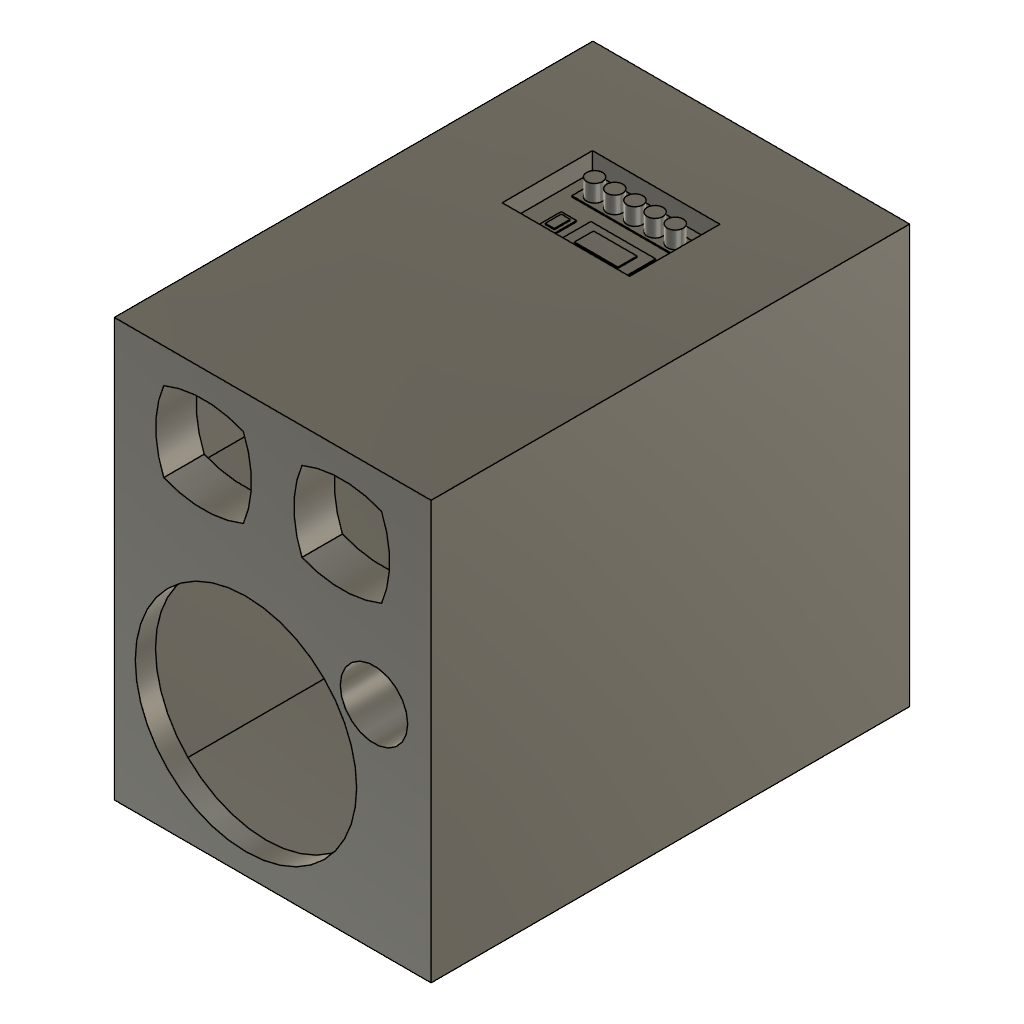
Speaker (Autodesk Fusion 360 design; units mm, degrees)
Autodesk Fusion 360 part; units mm, degrees
sketch "Sketch1" plane through (0, 0, 0) normal (0, 0, 1) x (1, 0, 0)
  line L0 (0, 0) -> (298.45, 0)
  line L1 (298.45, 0) -> (298.45, 450.85)
  line L2 (298.45, 450.85) -> (0, 450.85)
  line L3 (0, 450.85) -> (0, 0)
  dimension "d1" = 298.45
  dimension "d2" = 450.85
  constraint horizontal L0
  constraint vertical L1
  constraint horizontal L2
  constraint vertical L3
  constraint coincident L0.start L3.end
  measures "d1" distance of L0.start L0.end
  measures "d2" distance of L0.start L2.end
extrude "Extrude1" add sketch "Sketch1" along normal blind 254 makes body 1
sketch "Sketch2" plane through (0, 0, 0) normal (0, -1, 0) x (1, 0, 0)
  line L0 (0, 0) -> (298.45, 0)
  line L1 (298.45, 0) -> (298.45, 254)
  line L2 (298.45, 254) -> (0, 254)
  line L3 (0, 254) -> (0, 0)
  line L4 (19.05, 19.05) -> (279.4, 19.05)
  line L5 (279.4, 19.05) -> (279.4, 234.95)
  line L6 (279.4, 234.95) -> (19.05, 234.95)
  line L7 (19.05, 234.95) -> (19.05, 19.05)
  circle A0 centre (124.05, 124.05) radius 104.25
  circle A1 centre (244.65, 200.2) radius 31.75
  circle A2 centre (244.65, 200.2) radius 34.75
  dimension "d5" = -19.05
  dimension "d6" = 208.5
  dimension "d7" = 105
  dimension "d8" = 105
  dimension "d9" = 63.5
  dimension "d10" = 34.75
  dimension "d11" = 34.75
  dimension "d12" = 3
  measures "d6" diameter of A0
  measures "d7" distance of L7 A0.centre
  measures "d8" distance of L4 A0.centre
  measures "d9" diameter of A1
  measures "d10" distance of L5 A1.centre
  measures "d11" distance of L6 A1.centre
extrude "Extrude2" add 1 faces at (99.4833, 150.2833, 254) along direction (0, 0, 1) blind 139.7 on bodies 1 bodies 1
sketch "Sketch3" plane through (0, 0, 0) normal (0, -1, 0) x (1, 0, 0)
  line L0 (0, 0) -> (298.45, 0)
  line L1 (298.45, 0) -> (298.45, 393.7)
  line L2 (298.45, 393.7) -> (0, 393.7)
  line L3 (0, 393.7) -> (0, 0)
  line L4 (298.45, 254) -> (0, 254)
  line L5 (0, 393.7) -> (298.45, 393.7)
  line L6 (298.45, 393.7) -> (298.45, 254)
  line L7 (298.45, 254) -> (0, 254)
  line L8 (0, 254) -> (0, 393.7)
  line L9 (279.4, 273.05) -> (19.05, 273.05)
  line L10 (19.05, 273.05) -> (19.05, 374.65)
  line L11 (19.05, 374.65) -> (279.4, 374.65)
  line L12 (279.4, 374.65) -> (279.4, 273.05)
  line L13 (46.6375, 361.35) -> (121.6375, 361.35)
  line L14 (121.6375, 361.35) -> (121.6375, 286.35)
  line L15 (121.6375, 286.35) -> (46.6375, 286.35)
  line L16 (46.6375, 286.35) -> (46.6375, 361.35)
  line L17 (84.1375, 361.35) -> (84.1375, 340.8281)
  line L18 (19.05, 374.65) -> (149.225, 374.65)
  line L19 (149.225, 374.65) -> (279.4, 374.65)
  line L20 (46.6375, 323.85) -> (54.2725, 323.85)
  line L21 (149.225, 374.65) -> (149.225, 361.3588)
  arc A0 (121.6375, 361.35) -> (46.6375, 361.35) centre (84.1375, 271.8919) ccw
  arc A1 (46.6375, 286.35) -> (121.6375, 286.35) centre (84.1375, 375.8081) ccw
  arc A2 (121.6375, 286.35) -> (121.6375, 361.35) centre (32.1794, 323.85) ccw
  arc A3 (46.6375, 361.35) -> (46.6375, 286.35) centre (136.0956, 323.85) ccw
  arc A4 (251.8125, 361.35) -> (176.8125, 361.35) centre (214.3125, 271.8919) ccw
  arc A5 (176.8125, 361.35) -> (176.8125, 286.35) centre (266.2706, 323.85) ccw
  arc A6 (176.8125, 286.35) -> (251.8125, 286.35) centre (214.3125, 375.8081) ccw
  arc A7 (251.8125, 286.35) -> (251.8125, 361.35) centre (162.3544, 323.85) ccw
  dimension "d15" = 19.05
  dimension "d16" = 75
  dimension "d17" = 75
  dimension "d18" = 65.0875
  dimension "d19" = 50.8
  dimension "d20" = 97
  dimension "d21" = 97
  dimension "d22" = 97
  dimension "d23" = 97
  constraint horizontal L5
  constraint vertical L6
  constraint horizontal L7
  constraint vertical L8
  constraint coincident L4.start L6.end
  constraint coincident L2.end L3.start
  constraint horizontal L13
  constraint vertical L14
  constraint horizontal L15
  constraint vertical L16
  constraint midpoint L13 L17.start
  constraint perpendicular L13 L17
  constraint midpoint L11 L18.end
  constraint midpoint L16 L20.start
  constraint perpendicular L16 L20
  constraint perpendicular L11 L21
  constraint symmetric L13.start L21 A4.start
  constraint symmetric L13.end L21 A4.end
  constraint symmetric L14.end L21 A5.end
  constraint symmetric L15.end L21 A6.end
  constraint symmetric L21 A0 A4
  constraint symmetric L21 A1 A6
  constraint symmetric L21 A2 A5
  constraint symmetric L21 A3 A7
  measures "d16" distance of L13.start L13.end
  measures "d17" distance of L13.start L15.end
  measures "d18" distance of L10 L17
  measures "d19" distance of L18 L20
  measures "d20" radius of A0
  measures "d21" radius of A2
  measures "d22" radius of A1
  measures "d23" radius of A3
extrude "Extrude3" cut sketch "Sketch3" sketch "Sketch2" against normal blind 19.05 contours L13 A0 | L13 L14 L15 L16 | L16 A3 | L14 A2 | L15 A1 | A4 A5 A6 A7 of sketch 2 contours A0 bodies 1
shell "Shell1" thickness 19.05 removed faces 1 at (78.1482, 19.05, 149.2169) on bodies 1
extrude "Extrude4" cut 1 faces at (69.1235, 19.05, 323.85) along direction (0, 1, 0) blind 45 on bodies 1 bodies 1
extrude "Extrude5" cut 1 faces at (214.3125, 19.05, 308.836) along direction (0, 1, 0) blind 95 on bodies 1 bodies 1
extrude "Extrude6" add sketch "Sketch2" against normal blind 314.96 contours A2 | A1 bodies 1
extrude "Extrude7" cut sketch "Sketch2" against normal blind 325 contours A1 bodies 1
sketch "Sketch4" plane through (298.45, 0, 0) normal (1, 0, 0) x (0, 1, 0)
  line L0 (0, 0) -> (450.85, 0)
  line L1 (450.85, 0) -> (450.85, 393.7)
  line L2 (450.85, 393.7) -> (0, 393.7)
  line L3 (0, 393.7) -> (0, 0)
  line L4 (0, 254) -> (263.525, 254)
  line L5 (263.525, 254) -> (450.85, 254)
  line L6 (450.85, 254) -> (450.85, 393.7)
  line L7 (450.85, 393.7) -> (263.525, 393.7)
  line L8 (263.525, 393.7) -> (263.525, 254)
  point P0 (0, 254)
  dimension "d35" = 263.525
  constraint coincident P0 L4.start
  constraint perpendicular L3 L4
  constraint horizontal L5
  constraint vertical L6
  constraint horizontal L7
  constraint vertical L8
  constraint coincident L1.end L2.start
  measures "d35" distance of P0 L4.end
extrude "Extrude8" cut sketch "Sketch4" against normal blind 390 contours L1 L2 L5 L6 L7 L8 bodies 1
sketch "Sketch5" plane through (0, 450.85, 0) normal (0, 1, 0) x (-1, 0, 0)
  line L0 (0, 254) -> (-298.45, 254)
  line L1 (-298.45, 254) -> (-298.45, 0)
  line L2 (-298.45, 0) -> (0, 0)
  line L3 (0, 0) -> (0, 254)
  line L4 (-298.45, 254) -> (0, 254)
  line L5 (0, 254) -> (0, 234.95)
  line L6 (0, 234.95) -> (-298.45, 234.95)
  line L7 (-298.45, 234.95) -> (-298.45, 254)
  dimension "d38" = 19.05
  constraint horizontal L4
  constraint vertical L5
  constraint horizontal L6
  constraint vertical L7
  constraint coincident L0.end L1.start
  measures "d38" distance of L0.end L6.end
extrude "Extrude9" add sketch "Sketch5" against normal blind 450 contours L0 L1 L3 L4 L5 L6 L7 bodies 1
sketch "Sketch6" plane through (0, 0, 393.7) normal (0, 0, 1) x (-1, 0, 0)
  line L0 (-298.45, -263.525) -> (0, -263.525)
  line L1 (0, -263.525) -> (0, 0)
  line L2 (0, 0) -> (-298.45, 0)
  line L3 (-298.45, 0) -> (-298.45, -263.525)
  line L4 (0, -263.525) -> (-298.45, -263.525)
  line L5 (-298.45, -263.525) -> (-298.45, -244.475)
  line L6 (-298.45, -244.475) -> (0, -244.475)
  line L7 (0, -244.475) -> (0, -263.525)
  dimension "d41" = 19.05
  constraint horizontal L4
  constraint vertical L5
  constraint horizontal L6
  constraint vertical L7
  constraint coincident L0.end L1.start
  measures "d41" distance of L0.end L6.end
extrude "Extrude10" add sketch "Sketch6" against normal blind 140 contours L0 L1 L3 L4 L5 L6 L7 bodies 1
sketch "Battery" plane through (0, 0, 254) normal (0, 0, 1) x (-1, 0, 0)
  line L0 (0, -263.525) -> (-298.45, -263.525)
  line L1 (-298.45, -263.525) -> (-298.45, -450.85)
  line L2 (-298.45, -450.85) -> (0, -450.85)
  line L3 (0, -450.85) -> (0, -263.525)
  line L4 (-217.7141, -363.1024) -> (-80.7141, -363.1024)
  line L5 (-80.7141, -363.1024) -> (-80.7141, -429.8524)
  line L6 (-80.7141, -429.8524) -> (-217.7141, -429.8524)
  line L7 (-217.7141, -429.8524) -> (-217.7141, -363.1024)
  line L8 (-198.0587, -450.85) -> (-198.0587, -431.8)
  dimension "d44" = 137
  dimension "d45" = 66.75
  dimension "d100" = 19.05
  constraint horizontal L4
  constraint vertical L5
  constraint horizontal L6
  constraint vertical L7
  constraint coincident L2 L8.start
  constraint perpendicular L2 L8
  measures "d44" distance of L4.start L4.end
  measures "d45" distance of L4.start L6.end
  measures "d100" distance of L8.start L8.end
extrude "Extrude11" add sketch "Battery" along normal blind 82 separate body contours L4 L5 L6 L7 makes body 2
sketch "Sketch8" plane through (0, 0, 254) normal (0, 0, 1) x (-1, 0, 0)
  line L0 (0, -263.525) -> (-298.45, -263.525)
  line L1 (-298.45, -263.525) -> (-298.45, -450.85)
  line L2 (-298.45, -450.85) -> (0, -450.85)
  line L3 (0, -450.85) -> (0, -263.525)
  line L4 (-298.45, -450.85) -> (0, -450.85)
  line L5 (0, -450.85) -> (0, -431.8)
  line L6 (0, -431.8) -> (-298.45, -431.8)
  line L7 (-298.45, -431.8) -> (-298.45, -450.85)
  dimension "d48" = 19.05
  constraint horizontal L4
  constraint vertical L5
  constraint horizontal L6
  constraint vertical L7
  constraint coincident L1.end L2.start
  measures "d48" distance of L1.end L6.end
extrude "Extrude12" add sketch "Sketch8" along normal blind 139.7 separate body contours L1 L2 L3 L4 L5 L6 L7 makes body 3
sketch "Sketch9" plane through (0, 263.525, 0) normal (0, 1, 0) x (-1, 0, 0)
  line L0 (0, 254) -> (0, 393.7)
  line L1 (0, 393.7) -> (-298.45, 393.7)
  line L2 (-298.45, 393.7) -> (-298.45, 254)
  line L3 (-298.45, 254) -> (0, 254)
  line L4 (-279.4, 273.05) -> (-19.05, 273.05)
  line L5 (-19.05, 273.05) -> (-19.05, 374.65)
  line L6 (-19.05, 374.65) -> (-279.4, 374.65)
  line L7 (-279.4, 374.65) -> (-279.4, 273.05)
  line L8 (-279.4, 273.05) -> (-279.4, 254)
  line L9 (-19.05, 273.05) -> (-19.05, 254)
  dimension "d51" = -19.05
  constraint coincident L3 L8.end
  constraint perpendicular L3 L8
  constraint coincident L3 L9.end
  constraint perpendicular L3 L9
extrude "Extrude13" add sketch "Sketch9" along normal blind 168.275 contours L0 L1 L2 L3 L5 L6 L7 L8 L9 bodies 3 2 1
ref_plane "WorkPlane1" through (0, 0, 373.7) normal (0, 0, 1) x (1, 0, 0)
ref_plane "WorkPlane2" through (0, 430.85, 0) normal (0, 1, 0) x (0, 0, 1)
sketch "Sketch10" plane through (0, 0, 393.7) normal (0, 0, 1) x (-1, 0, 0)
  line L0 (-298.45, 0) -> (-298.45, -450.85)
  line L1 (-298.45, -450.85) -> (0, -450.85)
  line L2 (0, -450.85) -> (0, 0)
  line L3 (0, 0) -> (-298.45, 0)
  line L4 (-279.4, -263.525) -> (-19.05, -263.525)
  line L5 (-19.05, -263.525) -> (-279.4, -263.525)
  line L6 (-149.225, -263.525) -> (-149.225, -276.225)
  line L7 (-149.225, -276.225) -> (-209.225, -276.225)
  line L8 (-209.225, -276.225) -> (-89.225, -276.225)
  line L9 (-89.225, -276.225) -> (-89.225, -361.225)
  line L10 (-89.225, -361.225) -> (-209.225, -361.225)
  line L11 (-209.225, -361.225) -> (-209.225, -276.225)
  line L12 (-212.725, -272.725) -> (-85.725, -272.725)
  line L13 (-85.725, -272.725) -> (-85.725, -364.725)
  line L14 (-85.725, -364.725) -> (-212.725, -364.725)
  line L15 (-212.725, -364.725) -> (-212.725, -272.725)
  dimension "d56" = 12.7
  dimension "d57" = 60
  dimension "d58" = 120
  dimension "d59" = 85
  dimension "d60" = -3.5
  constraint midpoint L4 L6.start
  constraint perpendicular L4 L6
  constraint perpendicular L6 L7
  constraint horizontal L8
  constraint vertical L9
  constraint horizontal L10
  constraint vertical L11
  measures "d56" distance of L6.start L6.end
  measures "d57" distance of L6.end L7.end
  measures "d58" distance of L7.end L8.end
  measures "d59" distance of L7.end L10.end
extrude "Extrude14" cut sketch "Sketch10" against normal blind 30 contours L7 L8 L9 L10 L11 bodies 3
extrude "Extrude15" add sketch "Sketch10" against normal blind 21 contours L12 L13 L14 L15 bodies 3
sketch "Sketch11" plane through (0, 276.225, 0) normal (0, 1, 0) x (-1, 0, 0)
  line L0 (-89.225, 372.7) -> (-89.225, 393.7)
  line L1 (-89.225, 393.7) -> (-209.225, 393.7)
  line L2 (-209.225, 393.7) -> (-209.225, 372.7)
  line L3 (-209.225, 372.7) -> (-89.225, 372.7)
  line L4 (-209.225, 372.7) -> (-89.225, 372.7)
  line L5 (-89.225, 372.7) -> (-89.225, 376.2)
  line L6 (-89.225, 376.2) -> (-209.225, 376.2)
  line L7 (-209.225, 376.2) -> (-209.225, 372.7)
  dimension "d65" = 3.5
  constraint horizontal L4
  constraint vertical L5
  constraint horizontal L6
  constraint vertical L7
  constraint coincident L2.end L3.start
  measures "d65" distance of L2.end L6.end
extrude "Extrude16" add sketch "Sketch11" along normal blind 85 separate body contours L0 L2 L3 L4 L5 L6 L7 makes body 4
sketch "Sketch12" plane through (0, 0, 376.2) normal (0, 0, 1) x (-1, 0, 0)
  line L0 (-89.225, -276.225) -> (-209.225, -276.225)
  line L1 (-209.225, -276.225) -> (-209.225, -361.225)
  line L2 (-209.225, -361.225) -> (-89.225, -361.225)
  line L3 (-89.225, -361.225) -> (-89.225, -276.225)
  line L4 (-198.725, -331.225) -> (-99.725, -331.225)
  line L5 (-99.725, -331.225) -> (-99.725, -351.225)
  line L6 (-99.725, -351.225) -> (-198.725, -351.225)
  line L7 (-198.725, -351.225) -> (-198.725, -331.225)
  line L8 (-190.725, -286.225) -> (-129.725, -286.225)
  line L9 (-129.725, -286.225) -> (-129.725, -319.225)
  line L10 (-129.725, -319.225) -> (-190.725, -319.225)
  line L11 (-190.725, -319.225) -> (-190.725, -286.225)
  line L12 (-122.225, -292.225) -> (-107.725, -292.225)
  line L13 (-107.725, -292.225) -> (-107.725, -313.225)
  line L14 (-107.725, -313.225) -> (-122.225, -313.225)
  line L15 (-122.225, -313.225) -> (-122.225, -292.225)
  line L16 (-107.725, -302.725) -> (-107.7476, -302.725)
  circle A0 centre (-149.225, -341.225) radius 7.5
  circle A1 centre (-130.225, -341.225) radius 7.5
  circle A2 centre (-111.225, -341.225) radius 7.5
  circle A3 centre (-168.225, -341.225) radius 7.5
  circle A4 centre (-187.225, -341.225) radius 7.5
  line L17 (-190.725, -286.225) -> (-180.725, -286.225)
  line L18 (-180.725, -286.225) -> (-180.725, -293.725)
  line L19 (-180.725, -293.725) -> (-190.725, -293.725)
  line L20 (-190.725, -293.725) -> (-190.725, -286.225)
  line L21 (-180.725, -293.725) -> (-139.725, -293.725)
  line L22 (-139.725, -293.725) -> (-139.725, -311.725)
  line L23 (-139.725, -311.725) -> (-180.725, -311.725)
  line L24 (-180.725, -311.725) -> (-180.725, -293.725)
  line L25 (-110.725, -310.225) -> (-119.225, -310.225)
  line L26 (-119.225, -310.225) -> (-119.225, -295.225)
  line L27 (-119.225, -295.225) -> (-110.725, -295.225)
  line L28 (-110.725, -295.225) -> (-110.725, -310.225)
  dimension "d68" = 99
  dimension "d69" = 20
  dimension "d70" = 10.5
  dimension "d71" = 10.5
  dimension "d72" = 61
  dimension "d73" = 33
  dimension "d74" = 14.5
  dimension "d75" = 21
  dimension "d76" = 8
  dimension "d77" = 8
  dimension "d78" = 16.5
  dimension "d79" = 10
  dimension "d80" = 10
  dimension "d81" = 12
  dimension "d82" = 15
  dimension "d83" = 15
  dimension "d84" = 15
  dimension "d85" = 19
  dimension "d86" = 38
  dimension "d87" = 15
  dimension "d88" = 15
  dimension "d89" = 19
  dimension "d90" = 38
  dimension "d91" = 10
  dimension "d92" = 7.5
  dimension "d93" = 41
  dimension "d94" = 18
  dimension "d95" = 3
  constraint horizontal L4
  constraint vertical L5
  constraint horizontal L6
  constraint vertical L7
  constraint horizontal L8
  constraint vertical L9
  constraint horizontal L10
  constraint vertical L11
  constraint horizontal L12
  constraint vertical L13
  constraint horizontal L14
  constraint vertical L15
  constraint midpoint L13 L16.start
  constraint perpendicular L13 L16
  constraint horizontal L17
  constraint vertical L18
  constraint horizontal L19
  constraint vertical L20
  constraint horizontal L21
  constraint vertical L22
  constraint horizontal L23
  constraint vertical L24
  measures "d68" distance of L4.start L4.end
  measures "d69" distance of L4.start L6.end
  measures "d70" distance of L1 L7
  measures "d71" distance of L3 L5
  measures "d72" distance of L8.start L8.end
  measures "d73" distance of L8.start L10.end
  measures "d74" distance of L12.start L12.end
  measures "d75" distance of L12.start L14.end
  measures "d76" distance of L5 L13
  measures "d77" distance of L7 L11
  measures "d78" distance of L8 L16
  measures "d79" distance of L0 L8
  measures "d80" distance of L2 L6
  measures "d81" distance of L4 L10
  measures "d82" diameter of A0
  measures "d83" diameter of A1
  measures "d84" diameter of A2
  measures "d85" distance of A0.centre A1.centre
  measures "d86" distance of A0.centre A2.centre
  measures "d87" diameter of A3
  measures "d88" diameter of A4
  measures "d89" distance of A0.centre A3.centre
  measures "d90" distance of A0.centre A4.centre
  measures "d91" distance of L8.start L17.end
  measures "d92" distance of L8.start L19.end
  measures "d93" distance of L18.end L21.end
  measures "d94" distance of L18.end L23.end
extrude "Extrude17" add sketch "Sketch12" along normal blind 2 contours L21 L22 L23 L24 | A0 | A1 | A2 | A3 | A4 | L25 L26 L27 L28 bodies 4
extrude "Extrude18" add sketch "Sketch12" along normal blind 1 contours L4 L5 L6 L7 | L8 L11 L17 L18 L19 L20 | L8 L9 L10 L11 L18 L19 | L12 L13 L14 L15 bodies 4
sketch "Sketch13" plane through (0, 0, 372.7) normal (0, 0, -1) x (1, 0, 0)
  line L0 (209.225, -276.225) -> (89.225, -276.225)
  line L1 (89.225, -276.225) -> (89.225, -361.225)
  line L2 (89.225, -361.225) -> (209.225, -361.225)
  line L3 (209.225, -361.225) -> (209.225, -276.225)
  line L4 (99.725, -351.225) -> (198.725, -351.225)
  line L5 (198.725, -351.225) -> (198.725, -331.225)
  line L6 (198.725, -331.225) -> (99.725, -331.225)
  line L7 (99.725, -331.225) -> (99.725, -351.225)
  line L8 (198.725, -351.225) -> (99.725, -351.225)
  line L9 (99.725, -351.225) -> (99.725, -331.225)
  line L10 (99.725, -331.225) -> (198.725, -331.225)
  line L11 (198.725, -331.225) -> (198.725, -351.225)
  constraint horizontal L8
  constraint vertical L9
  constraint horizontal L10
  constraint vertical L11
  constraint coincident L6.end L7.start
  constraint coincident L4.end L5.start
extrude "Extrude19" add sketch "Sketch13" along normal blind 97.5 contours L4 L5 L6 L7 L8 L9 L10 L11 bodies 4
sketch "Sketch14" plane through (0, 0, 372.7) normal (0, 0, -1) x (1, 0, 0)
  line L0 (198.725, -331.225) -> (198.725, -351.225)
  line L1 (198.725, -351.225) -> (99.725, -351.225)
  line L2 (99.725, -351.225) -> (99.725, -331.225)
  line L3 (99.725, -331.225) -> (198.725, -331.225)
  line L4 (209.225, -276.225) -> (89.225, -276.225)
  line L5 (89.225, -276.225) -> (89.225, -361.225)
  line L6 (89.225, -361.225) -> (209.225, -361.225)
  line L7 (209.225, -361.225) -> (209.225, -276.225)
  line L8 (129.725, -319.225) -> (190.725, -319.225)
  line L9 (190.725, -286.225) -> (129.725, -286.225)
  line L10 (190.725, -319.225) -> (129.725, -319.225)
  line L11 (129.725, -319.225) -> (129.725, -286.225)
  line L12 (129.725, -286.225) -> (190.725, -286.225)
  line L13 (190.725, -286.225) -> (190.725, -319.225)
  constraint horizontal L10
  constraint vertical L11
  constraint horizontal L12
  constraint vertical L13
  constraint coincident L9.end L11.end
  constraint coincident L8.end L10.start
extrude "Extrude20" add sketch "Sketch14" along normal blind 10.5 contours L8 L9 L10 L11 L12 L13 bodies 4
sketch "Sketch15" plane through (0, 0, 372.7) normal (0, 0, -1) x (1, 0, 0)
  line L0 (190.725, -286.225) -> (190.725, -319.225)
  line L1 (190.725, -319.225) -> (129.725, -319.225)
  line L2 (129.725, -319.225) -> (129.725, -286.225)
  line L3 (129.725, -286.225) -> (190.725, -286.225)
  line L4 (198.725, -331.225) -> (198.725, -351.225)
  line L5 (198.725, -351.225) -> (99.725, -351.225)
  line L6 (99.725, -351.225) -> (99.725, -331.225)
  line L7 (99.725, -331.225) -> (198.725, -331.225)
  line L8 (209.225, -276.225) -> (89.225, -276.225)
  line L9 (89.225, -276.225) -> (89.225, -361.225)
  line L10 (89.225, -361.225) -> (209.225, -361.225)
  line L11 (209.225, -361.225) -> (209.225, -276.225)
  line L12 (107.725, -313.225) -> (122.225, -313.225)
  line L13 (122.225, -292.225) -> (107.725, -292.225)
  line L14 (122.225, -313.225) -> (107.725, -313.225)
  line L15 (107.725, -313.225) -> (107.725, -292.225)
  line L16 (107.725, -292.225) -> (122.225, -292.225)
  line L17 (122.225, -292.225) -> (122.225, -313.225)
  constraint horizontal L14
  constraint vertical L15
  constraint horizontal L16
  constraint vertical L17
  constraint coincident L13.end L15.end
  constraint coincident L12.end L14.start
extrude "Extrude21" add sketch "Sketch15" along normal blind 11 contours L12 L13 L14 L15 L16 L17 bodies 4
extrude "Extrude22" add 5 faces at (185.6663, 342.6713, 378.2) (171.9142, 339.8123, 378.2) (147.3924, 339.5246, 378.2) (131.1663, 339.2704, 378.2) (109.6663, 343.1796, 378.2) along direction (0, 0, 1) blind 15 on bodies 4 bodies 4
sketch "Sketch16" plane through (0, 0, 0) normal (0, -1, 0) x (1, 0, 0)
  circle A0 centre (244.65, 200.2) radius 31.75
  arc A1 (251.8125, 361.35) -> (176.8125, 361.35) centre (214.3125, 271.8919) ccw
  arc A2 (251.8125, 286.35) -> (251.8125, 361.35) centre (162.3544, 323.85) ccw
  arc A3 (176.8125, 286.35) -> (251.8125, 286.35) centre (214.3125, 375.8081) ccw
  arc A4 (176.8125, 361.35) -> (176.8125, 286.35) centre (266.2706, 323.85) ccw
  arc A5 (46.6375, 286.35) -> (121.6375, 286.35) centre (84.1375, 375.8081) ccw
  arc A6 (46.6375, 361.35) -> (46.6375, 286.35) centre (136.0956, 323.85) ccw
  arc A7 (121.6375, 361.35) -> (46.6375, 361.35) centre (84.1375, 271.8919) ccw
  arc A8 (121.6375, 286.35) -> (121.6375, 361.35) centre (32.1794, 323.85) ccw
  circle A9 centre (124.05, 124.05) radius 104.25
  line L0 (0, 0) -> (298.45, 0)
  line L1 (298.45, 0) -> (298.45, 393.7)
  line L2 (298.45, 393.7) -> (0, 393.7)
  line L3 (0, 393.7) -> (0, 0)
  circle A10 centre (124.05, 124.05) radius 88.5
  dimension "d109" = 177
  constraint concentric A9 A10
  measures "d109" diameter of A10
ref_plane "WorkPlane3" through (149.225, 40, 196.85) normal (0, -1, 0) x (1, 0, 0)
equation "d8 = d7"
equation "d10 = ( ( 63.5 / 2 ) * 1 mm ) + 3 mm"
equation "d11 = d10"
equation "d18 = ( 130.175 / 2 ) * 1 mm"
equation "d19 = ( 101.6 / 2 ) * 1 mm"
equation "d59 = 64 mm + 21 mm"
equation "d78 = ( 33 / 2 ) * 1 mm"
equation "d86 = ( 19 * 2 ) * 1 mm"
equation "d89 = d85"
equation "d90 = d86"
equation "d94 = 33 mm - 15 mm"
